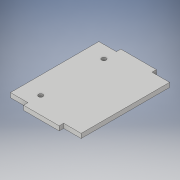
# Autodesk Inventor part: top
Saved by Autodesk Inventor 2017 (Build 210142000, 142)
## iProperties
Created: 2017-06-27
Part Number: top
Material: Generic
Document SubType Name: Modeling
Designer: millerid
Density: 1 g/cm^3
Appearance: Default
Author: millerid
Autodesk Inventor part; units mm, degrees
ref_plane "YZ Plane" through (0, 0, 0) normal (1, 0, 0) x (0, 1, 0)
ref_plane "XZ Plane" through (0, 0, 0) normal (0, 1, 0) x (-1, 0, 0)
ref_plane "XY Plane" through (0, 0, 0) normal (0, 0, 1) x (1, 0, 0)
sketch "Sketch1" plane through (0, 0, 0) normal (0, 1, 0) x (-1, 0, 0)
  line L0 (0, 0) -> (12.5984, 0)
  line L1 (12.5984, 0) -> (12.5984, 3.175)
  line L2 (12.5984, 3.175) -> (38.2016, 3.175)
  line L3 (38.2016, 3.175) -> (38.2016, 0)
  line L4 (38.2016, 0) -> (50.8, 0)
  line L5 (50.8, 0) -> (50.8, -63.5)
  line L6 (50.8, -63.5) -> (38.2016, -63.5)
  line L7 (38.2016, -63.5) -> (38.2016, -66.675)
  line L8 (38.2016, -66.675) -> (12.5984, -66.675)
  line L9 (12.5984, -66.675) -> (12.5984, -63.5)
  line L10 (12.5984, -63.5) -> (0, -63.5)
  line L11 (0, -63.5) -> (0, 0)
  circle A0 centre (38.1, -9.0551) radius 1.5875
  circle A1 centre (38.1, -54.4449) radius 1.5875
  dimension "d0" = 12.5984
  dimension "d1" = 3.175
  dimension "d2" = 25.6032
  dimension "d3" = 63.5
  dimension "d4" = 3.175
  dimension "d5" = 50.8
  dimension "d6" = 3.175
  dimension "d7" = 3.175
  dimension "d8" = 45.3898
  dimension "d9" = 12.7
  dimension "d10" = 9.0551
  constraints: 24 end point, 8 perpendicular, 4 point on line, 2 centre point, 2 collinear, 2 horizontal
  measures "d0" distance of L0.start L0.end
  measures "d1" distance of L0.end L1.end
  measures "d2" distance of L1.end L2.end
  measures "d3" distance of L4.end L5.end
  measures "d4" distance of L6.end L7.end
  measures "d5" distance between parallel lines of L5 L11
  measures "d6" diameter of A0
  measures "d7" diameter of A1
  measures "d8" distance of A1.centre A0.centre
  measures "d9" distance from line of L5 A1.centre
  measures "d10" distance from line of L6 A1.centre
extrude "Extrusion1" add sketch "Sketch1" along normal blind 3.175
equation "\"d10\" = -0.5 * d8 + 0.5 * d3"
body "Solid1"
